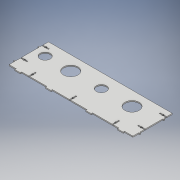
# Autodesk Inventor part: P1
Saved by Autodesk Inventor 2018 (Build 220112000, 112)
## iProperties
Created: 2018-02-28
Part Number: P1
Material: Generic
Document SubType Name: Modeling
Designer: isai
Density: 1 g/cm^3
Appearance: Default
Author: isai
Autodesk Inventor part; units mm, degrees
ref_plane "YZ Plane" through (0, 0, 0) normal (1, 0, 0) x (0, 1, 0)
sketch "Sketch2" plane through (0, 0, 0) normal (0, 0, 1) x (1, 0, 0)
  line L0 (220, -70) -> (-220, -70)
  line L1 (-220, -70) -> (-220, 70)
  line L2 (-220, 70) -> (220, 70)
  line L3 (220, 70) -> (220, -70)
  line L4 (220, -70) -> (-220, 70) construction
  line L5 (-220, -70) -> (220, 70) construction
  point P0 (0, 0)
  dimension "d8" = 440
  dimension "d9" = 140
  constraints: 12 end point, 2 midpoint, 2 parallel, 1 horizontal, 1 perpendicular
  measures "d8" distance of L1.end L2.end
  measures "d9" distance of L0.end L1.end
extrude "Extrusion2" add sketch "Sketch2" along normal blind 4
sketch "Sketch3" plane through (0, 0, 4) normal (0, 0, 1) x (1, 0, 0)
  line L0 (-220, -70) -> (220, -70) projected
  line L1 (220, -70) -> (220, 70) projected
  line L2 (220, 70) -> (-220, 70) projected
  line L3 (-220, 70) -> (-220, -70) projected
  circle A0 centre (-182, 20) radius 18
  circle A1 centre (-91, 20) radius 25.5
  circle A2 centre (18, 20) radius 18
  circle A3 centre (127, 20) radius 25.5
  point P0 (0, 0)
  dimension "d13" = 91
  dimension "d14" = 36
  dimension "d15" = 51
  dimension "d16" = 38
  dimension "d17" = 109
  dimension "d18" = 36
  dimension "d19" = 109
  dimension "d20" = 51
  dimension "d23" = 50
  constraints: 4 centre point, 2 coincident
  measures "d13" distance of A1.centre A0.centre
  measures "d14" diameter of A0
  measures "d15" diameter of A1
  measures "d16" distance from line of A0.centre L3
  measures "d17" distance of point (18, 20) A1.centre
  measures "d18" diameter of A2
  measures "d19" distance of point (127, 20) point (18, 20)
  measures "d20" diameter of A3
  measures "d23" distance from line of L2 A0.centre
extrude "Extrusion3" cut sketch "Sketch3" against normal blind 4 contours A0 | A1 | A2 | A3
sketch "Sketch4" plane through (0, 0, 4) normal (0, 0, 1) x (1, 0, 0)
  circle A0 centre (127, 20) radius 25.5
  circle A1 centre (18, 20) radius 25.5
  circle A2 centre (-91, 20) radius 18
  circle A3 centre (-182, 20) radius 18
  line L0 (-220, 70) -> (220, 70)
  line L1 (220, 70) -> (220, -70)
  line L2 (220, -70) -> (-220, -70)
  line L3 (-220, -70) -> (-220, 70)
  line L4 (220, 70) -> (224, 70)
  line L5 (224, -62.3) -> (220, -62.3)
  line L6 (224, 50) -> (197, 50)
  line L7 (197, 50) -> (197, 46.4)
  line L8 (197, 46.4) -> (224, 46.4)
  line L9 (224, 46.4) -> (224, 50)
  line L10 (210, 45.2) -> (207, 45.2)
  line L11 (207, 45.2) -> (207, 51.2)
  line L12 (207, 51.2) -> (210, 51.2)
  line L13 (210, 51.2) -> (210, 45.2)
  line L14 (210, 45.2) -> (207, 51.2) construction
  line L15 (207, 45.2) -> (210, 51.2) construction
  line L16 (224, -26.4) -> (197, -26.4)
  line L17 (197, -26.4) -> (197, -30)
  line L18 (197, -30) -> (224, -30)
  line L19 (224, -30) -> (224, -26.4)
  line L20 (210, -31.2) -> (207, -31.2)
  line L21 (207, -31.2) -> (207, -25.2)
  line L22 (207, -25.2) -> (210, -25.2)
  line L23 (210, -25.2) -> (210, -31.2)
  line L24 (210, -31.2) -> (207, -25.2) construction
  line L25 (207, -31.2) -> (210, -25.2) construction
  line L26 (224, 70) -> (224, 46.4)
  line L27 (224, -26.4) -> (224, -30)
  line L28 (220, -62.3) -> (220, -30)
  point P0 (0, 0)
  point P1 (208.5, 48.2)
  point P2 (208.5, -28.2)
  point P3 (220, 46.4)
  point P4 (220, -26.4)
  dimension "d24" = 4
  dimension "d25" = 27
  dimension "d26" = 3.6
  dimension "d27" = 3
  dimension "d28" = 6
  dimension "d29" = 10
  dimension "d30" = 140
  dimension "d31" = 20
  dimension "d32" = 27
  dimension "d33" = 3
  dimension "d34" = 6
  dimension "d35" = 40
  dimension "d36" = 3.6
  constraints: 58 end point, 11 parallel, 6 perpendicular, 5 horizontal, 4 centre point, 4 midpoint, 4 point on line
  measures "d24" distance of L5.start L28.start
  measures "d25" distance of L8.end L7.end
  measures "d26" distance of L7.end L6.end
  measures "d27" distance of L11.end L12.end
  measures "d28" distance of L10.end L11.end
  measures "d29" distance between parallel lines of L1 L13
  measures "d30" distance between parallel lines of L2 L0
  measures "d31" distance between parallel lines of L6 L0
  measures "d32" distance of L18.end L17.end
  measures "d33" distance of L22.start L22.end
  measures "d34" distance of L21.start L22.start
  measures "d35" distance between parallel lines of L2 L18
  measures "d36" distance of L17.start L17.end
extrude "Extrusion4" cut sketch "Sketch4" against normal blind 4 contours L6 L9 L8 L1 | L1 L8 L13 L6 | L13 L8 L11 L6 | L6 L11 L12 L13 | L16 L19 L18 L1 | L1 L18 L23 L16 | L13 L10 L11 L8 | L11 L8 L7 L6 | L23 L18 L21 L16 | L16 L21 L22 L23 | L23 L20 L21 L18 | L21 L18 L17 L16
ref_plane "Work Plane1" through (0, 70, 4) normal (1, 0, 0) x (0, 0, -1)
mirror "Mirror1" about plane through (0, 70, 4) normal (1, 0, 0) of "Extrusion4"
sketch "Sketch5" plane through (0, 0, 4) normal (0, 0, 1) x (1, 0, 0)
  line L0 (-224, -46) -> (-220, -46)
  line L1 (-224, -50) -> (-224, -46)
  line L2 (-220, -50) -> (-224, -50)
  line L3 (-220, -50) -> (-220, -70)
  line L4 (-220, -70) -> (220, -70)
  line L5 (220, -70) -> (220, -50)
  line L6 (220, -50) -> (224, -50)
  line L7 (224, -50) -> (224, -46)
  line L8 (224, -46) -> (220, -46)
  line L9 (-150, -57) -> (-150, -47)
  line L10 (-151.2, -57) -> (-150, -57)
  line L11 (-150, -47) -> (-146.4, -47)
  line L12 (-146.4, -47) -> (-146.4, -57)
  line L13 (-146.4, -57) -> (-145.2, -57)
  line L14 (-150, -60) -> (-151.2, -60)
  line L15 (-151.2, -60) -> (-151.2, -57)
  line L16 (-145.2, -57) -> (-145.2, -60)
  line L17 (-145.2, -60) -> (-146.4, -60)
  line L18 (-150, -70) -> (-150, -60)
  line L19 (-146.4, -60) -> (-146.4, -70)
  line L20 (-146.4, -70) -> (-150, -70)
  line L21 (-220, -70) -> (220, -70)
  line L22 (151.2, -57) -> (151.2, -60)
  line L23 (150, -57) -> (151.2, -57)
  line L24 (150, -47) -> (150, -57)
  line L25 (146.4, -47) -> (150, -47)
  line L26 (150, -60) -> (150, -70)
  line L27 (146.4, -57) -> (146.4, -47)
  line L28 (146.4, -70) -> (146.4, -60)
  line L29 (145.2, -57) -> (146.4, -57)
  line L30 (145.2, -60) -> (145.2, -57)
  line L31 (146.4, -60) -> (145.2, -60)
  line L32 (151.2, -60) -> (150, -60)
  line L33 (150, -70) -> (146.4, -70)
  line L34 (-0.6, -57) -> (-0.6, -60)
  line L35 (-1.8, -57) -> (-0.6, -57)
  line L36 (-1.8, -47) -> (-1.8, -57)
  line L37 (-5.4, -47) -> (-1.8, -47)
  line L38 (-1.8, -60) -> (-1.8, -70)
  line L39 (-5.4, -57) -> (-5.4, -47)
  line L40 (-5.4, -70) -> (-5.4, -60)
  line L41 (-6.6, -57) -> (-5.4, -57)
  line L42 (-6.6, -60) -> (-6.6, -57)
  line L43 (-5.4, -60) -> (-6.6, -60)
  line L44 (-0.6, -60) -> (-1.8, -60)
  line L45 (-1.8, -70) -> (-5.4, -70)
  line L46 (-220, -70) -> (220, -70) projected
  point P0 (0, 0)
  point P1 (-143.2198, -70)
  point P2 (176.1378, -65.3908)
  point P3 (10.9651, -65.3908)
  dimension "d39" = 70
  dimension "d40" = 3.6
  dimension "d41" = 3.6
  dimension "d42" = 6
  dimension "d43" = 1.2
  dimension "d44" = 3
  dimension "d45" = 1.2
  dimension "d46" = 3.6
  dimension "d47" = 3.6
  dimension "d48" = 6
  dimension "d49" = 1.2
  dimension "d50" = 3
  dimension "d51" = 1.2
  dimension "d52" = 3.6
  dimension "d53" = 3.6
  dimension "d54" = 6
  dimension "d55" = 1.2
  dimension "d56" = 3
  dimension "d57" = 1.2
  dimension "d58" = 70
  dimension "d59" = 440
  dimension "d60" = 221.8
  constraints: 92 end point, 18 perpendicular, 3 parallel, 1 point on line
  measures "d39" distance between parallel lines of L18 L3
  measures "d40" distance between parallel lines of L19 L18
  measures "d41" distance between parallel lines of L12 L9
  measures "d42" distance between parallel lines of L16 L15
  measures "d43" distance between parallel lines of L15 L9
  measures "d44" distance between parallel lines of L14 L10
  measures "d45" distance between parallel lines of L18 L15
  measures "d46" distance between parallel lines of L26 L28
  measures "d47" distance between parallel lines of L24 L27
  measures "d48" distance between parallel lines of L22 L30
  measures "d49" distance between parallel lines of L30 L27
  measures "d50" distance between parallel lines of L31 L29
  measures "d51" distance between parallel lines of L28 L30
  measures "d52" distance between parallel lines of L38 L40
  measures "d53" distance between parallel lines of L36 L39
  measures "d54" distance between parallel lines of L34 L42
  measures "d55" distance between parallel lines of L42 L39
  measures "d56" distance between parallel lines of L43 L41
  measures "d57" distance between parallel lines of L40 L42
  measures "d58" distance between parallel lines of L5 L26
  measures "d59" distance between parallel lines of L5 L3
  measures "d60" distance between parallel lines of L5 L38
extrude "Extrusion5" cut sketch "Sketch5" against normal blind 10
sketch "Sketch6" plane through (0, 0, 4) normal (0, 0, 1) x (1, 0, 0)
  line L0 (-220, -70) -> (-150, -70)
  line L1 (-195, -70) -> (-175, -70)
  line L2 (-175, -70) -> (-175, -75)
  line L3 (-175, -75) -> (-195, -75)
  line L4 (-195, -75) -> (-195, -70)
  line L5 (-146.4, -70) -> (-5.4, -70)
  line L6 (-85.9, -70) -> (-65.9, -70)
  line L7 (-65.9, -70) -> (-65.9, -75)
  line L8 (-65.9, -75) -> (-85.9, -75)
  line L9 (-85.9, -75) -> (-85.9, -70)
  line L10 (-1.8, -70) -> (146.4, -70)
  line L11 (57.1516, -70) -> (77.1516, -70)
  line L12 (77.1516, -70) -> (77.1516, -75)
  line L13 (77.1516, -75) -> (57.1516, -75)
  line L14 (57.1516, -75) -> (57.1516, -70)
  line L15 (150, -70) -> (220, -70)
  line L16 (170.4397, -70) -> (190.4397, -70)
  line L17 (190.4397, -70) -> (190.4397, -75)
  line L18 (190.4397, -75) -> (170.4397, -75)
  line L19 (170.4397, -75) -> (170.4397, -70)
  line L20 (-220, -50) -> (-220, -70)
  line L21 (-146.4, -60) -> (-146.4, -70)
  line L22 (-5.4, -70) -> (-5.4, -60)
  line L23 (146.4, -70) -> (146.4, -60)
  line L24 (-1.8, -60) -> (-1.8, -70)
  line L25 (-1.8, -60) -> (-1.8, -70) projected
  line L26 (-1.8, -70) -> (146.4, -70) projected
  line L27 (146.4, -70) -> (146.4, -60) projected
  line L28 (146.4, -60) -> (145.2, -60) projected
  line L29 (145.2, -60) -> (145.2, -57) projected
  line L30 (145.2, -57) -> (146.4, -57) projected
  line L31 (146.4, -57) -> (146.4, -47) projected
  line L32 (146.4, -47) -> (150, -47) projected
  line L33 (150, -47) -> (150, -57) projected
  line L34 (150, -57) -> (151.2, -57) projected
  line L35 (151.2, -57) -> (151.2, -60) projected
  line L36 (151.2, -60) -> (150, -60) projected
  line L37 (150, -60) -> (150, -70) projected
  line L38 (150, -70) -> (220, -70) projected
  line L39 (220, -70) -> (220, -30) projected
  line L40 (220, -30) -> (210, -30) projected
  line L41 (210, -30) -> (210, -31.2) projected
  line L42 (210, -31.2) -> (207, -31.2) projected
  line L43 (207, -31.2) -> (207, -30) projected
  line L44 (207, -30) -> (197, -30) projected
  line L45 (197, -30) -> (197, -26.4) projected
  line L46 (197, -26.4) -> (207, -26.4) projected
  line L47 (207, -26.4) -> (207, -25.2) projected
  line L48 (207, -25.2) -> (210, -25.2) projected
  line L49 (210, -25.2) -> (210, -26.4) projected
  line L50 (210, -26.4) -> (220, -26.4) projected
  line L51 (220, -26.4) -> (220, 46.4) projected
  line L52 (220, 46.4) -> (210, 46.4) projected
  line L53 (210, 46.4) -> (210, 45.2) projected
  line L54 (210, 45.2) -> (207, 45.2) projected
  line L55 (207, 45.2) -> (207, 46.4) projected
  line L56 (207, 46.4) -> (197, 46.4) projected
  line L57 (197, 46.4) -> (197, 50) projected
  line L58 (197, 50) -> (207, 50) projected
  line L59 (207, 50) -> (207, 51.2) projected
  line L60 (207, 51.2) -> (210, 51.2) projected
  line L61 (210, 51.2) -> (210, 50) projected
  line L62 (210, 50) -> (220, 50) projected
  line L63 (220, 50) -> (220, 70) projected
  line L64 (220, 70) -> (-220, 70) projected
  line L65 (-220, 70) -> (-220, 50) projected
  line L66 (-220, 50) -> (-210, 50) projected
  line L67 (-210, 50) -> (-210, 51.2) projected
  line L68 (-210, 51.2) -> (-207, 51.2) projected
  line L69 (-207, 51.2) -> (-207, 50) projected
  line L70 (-207, 50) -> (-197, 50) projected
  line L71 (-197, 50) -> (-197, 46.4) projected
  line L72 (-197, 46.4) -> (-207, 46.4) projected
  line L73 (-207, 46.4) -> (-207, 45.2) projected
  line L74 (-207, 45.2) -> (-210, 45.2) projected
  line L75 (-210, 45.2) -> (-210, 46.4) projected
  line L76 (-210, 46.4) -> (-220, 46.4) projected
  line L77 (-220, 46.4) -> (-220, -26.4) projected
  line L78 (-220, -26.4) -> (-210, -26.4) projected
  line L79 (-210, -26.4) -> (-210, -25.2) projected
  line L80 (-210, -25.2) -> (-207, -25.2) projected
  line L81 (-207, -25.2) -> (-207, -26.4) projected
  line L82 (-207, -26.4) -> (-197, -26.4) projected
  line L83 (-197, -26.4) -> (-197, -30) projected
  line L84 (-197, -30) -> (-207, -30) projected
  line L85 (-207, -30) -> (-207, -31.2) projected
  line L86 (-207, -31.2) -> (-210, -31.2) projected
  line L87 (-210, -31.2) -> (-210, -30) projected
  line L88 (-210, -30) -> (-220, -30) projected
  line L89 (-220, -30) -> (-220, -70) projected
  line L90 (-220, -70) -> (-150, -70) projected
  line L91 (-150, -70) -> (-150, -60) projected
  line L92 (-150, -60) -> (-151.2, -60) projected
  line L93 (-151.2, -60) -> (-151.2, -57) projected
  line L94 (-151.2, -57) -> (-150, -57) projected
  line L95 (-150, -57) -> (-150, -47) projected
  line L96 (-150, -47) -> (-146.4, -47) projected
  line L97 (-146.4, -47) -> (-146.4, -57) projected
  line L98 (-146.4, -57) -> (-145.2, -57) projected
  line L99 (-145.2, -57) -> (-145.2, -60) projected
  line L100 (-145.2, -60) -> (-146.4, -60) projected
  line L101 (-146.4, -60) -> (-146.4, -70) projected
  line L102 (-146.4, -70) -> (-5.4, -70) projected
  line L103 (-5.4, -70) -> (-5.4, -60) projected
  line L104 (-5.4, -60) -> (-6.6, -60) projected
  line L105 (-6.6, -60) -> (-6.6, -57) projected
  line L106 (-6.6, -57) -> (-5.4, -57) projected
  line L107 (-5.4, -57) -> (-5.4, -47) projected
  line L108 (-5.4, -47) -> (-1.8, -47) projected
  line L109 (-1.8, -47) -> (-1.8, -57) projected
  line L110 (-1.8, -57) -> (-0.6, -57) projected
  line L111 (-0.6, -57) -> (-0.6, -60) projected
  line L112 (-0.6, -60) -> (-1.8, -60) projected
  circle A0 centre (-91, 20) radius 25.5 projected
  circle A1 centre (-182, 20) radius 18 projected
  circle A2 centre (18, 20) radius 18 projected
  circle A3 centre (127, 20) radius 25.5 projected
  line L113 (-220, -30) -> (-220, -70) projected
  point P0 (0, 0)
  dimension "d63" = 20
  dimension "d64" = 5
  dimension "d65" = 20
  dimension "d66" = 5
  dimension "d67" = 20
  dimension "d68" = 5
  dimension "d69" = 20
  dimension "d70" = 5
  dimension "d71" = 25
  dimension "d72" = 60.5
  dimension "d73" = 141
  dimension "d74" = 148.2
  constraints: 50 end point, 8 parallel, 4 horizontal, 4 perpendicular, 4 point on line, 2 coincident
  measures "d63" distance of L2.end L3.end
  measures "d64" distance of L2.start L2.end
  measures "d65" distance of L7.end L9.start
  measures "d66" distance of L6.end L7.end
  measures "d67" distance of L12.end L14.start
  measures "d68" distance of L12.start L12.end
  measures "d69" distance of L17.end L19.start
  measures "d70" distance of L17.start L17.end
  measures "d71" distance between parallel lines of L4 L20
  measures "d72" distance between parallel lines of L9 L21
  measures "d73" distance between parallel lines of L22 L21
  measures "d74" distance between parallel lines of L23 L24
extrude "Extrusion6" add sketch "Sketch6" against normal blind 4 contours L0 L2 L3 L4 | L5 L7 L8 L9 | L10 L12 L13 L14 | L15 L17 L18 L19
sketch "Sketch7" plane through (0, 0, 4) normal (0, 0, 1) x (1, 0, 0)
  line L0 (220, 70) -> (-220, 70)
  line L1 (210, -26.4) -> (220, -26.4)
  line L2 (220, -26.4) -> (220, 46.4)
  line L3 (220, 46.4) -> (210, 46.4)
  line L4 (210, 46.4) -> (210, 45.2)
  line L5 (210, 45.2) -> (207, 45.2)
  line L6 (207, 45.2) -> (207, 46.4)
  line L7 (207, 46.4) -> (197, 46.4)
  line L8 (197, 50) -> (207, 50)
  line L9 (207, 50) -> (207, 51.2)
  line L10 (207, 51.2) -> (210, 51.2)
  line L11 (210, 51.2) -> (210, 50)
  line L12 (210, 50) -> (220, 50)
  line L13 (220, 50) -> (220, 70)
  line L14 (220, 70) -> (-220, 70)
  line L15 (-220, -70) -> (220, -70)
  line L16 (220, -70) -> (220, -30)
  line L17 (220, -30) -> (210, -30)
  line L18 (210, -30) -> (210, -31.2)
  line L19 (210, -31.2) -> (207, -31.2)
  line L20 (207, -31.2) -> (207, -30)
  line L21 (207, -30) -> (197, -30)
  line L22 (197, -26.4) -> (207, -26.4)
  line L23 (207, -26.4) -> (207, -25.2)
  line L24 (207, -25.2) -> (210, -25.2)
  line L25 (210, -25.2) -> (210, -26.4)
  circle A0 centre (182, 20) radius 18
  line L26 (220, 40) -> (224, 40)
  line L27 (224, 40) -> (224, 36)
  line L28 (224, 36) -> (220, 36)
  line L29 (220, 36) -> (220, 40)
  line L30 (220, -46) -> (224, -46)
  line L31 (224, -46) -> (224, -50)
  line L32 (224, -50) -> (220, -50)
  line L33 (220, -50) -> (220, -46)
  line L34 (-1.8, -60) -> (-1.8, -70) projected
  line L35 (-1.8, -70) -> (57.1516, -70) projected
  line L36 (57.1516, -70) -> (57.1516, -75) projected
  line L37 (57.1516, -75) -> (77.1516, -75) projected
  line L38 (77.1516, -75) -> (77.1516, -70) projected
  line L39 (77.1516, -70) -> (146.4, -70) projected
  line L40 (146.4, -70) -> (146.4, -60) projected
  line L41 (146.4, -60) -> (145.2, -60) projected
  line L42 (145.2, -60) -> (145.2, -57) projected
  line L43 (145.2, -57) -> (146.4, -57) projected
  line L44 (146.4, -57) -> (146.4, -47) projected
  line L45 (146.4, -47) -> (150, -47) projected
  line L46 (150, -47) -> (150, -57) projected
  line L47 (150, -57) -> (151.2, -57) projected
  line L48 (151.2, -57) -> (151.2, -60) projected
  line L49 (151.2, -60) -> (150, -60) projected
  line L50 (150, -60) -> (150, -70) projected
  line L51 (150, -70) -> (170.4397, -70) projected
  line L52 (170.4397, -75) -> (170.4397, -70) projected
  line L53 (190.4397, -75) -> (170.4397, -75) projected
  line L54 (190.4397, -70) -> (190.4397, -75) projected
  line L55 (190.4397, -70) -> (220, -70) projected
  line L56 (220, -70) -> (220, -30) projected
  line L57 (220, -30) -> (210, -30) projected
  line L58 (210, -30) -> (210, -31.2) projected
  line L59 (210, -31.2) -> (207, -31.2) projected
  line L60 (207, -31.2) -> (207, -30) projected
  line L61 (207, -30) -> (197, -30) projected
  line L62 (197, -30) -> (197, -26.4) projected
  line L63 (197, -26.4) -> (207, -26.4) projected
  line L64 (207, -26.4) -> (207, -25.2) projected
  line L65 (207, -25.2) -> (210, -25.2) projected
  line L66 (210, -25.2) -> (210, -26.4) projected
  line L67 (210, -26.4) -> (220, -26.4) projected
  line L68 (220, -26.4) -> (220, 46.4) projected
  line L69 (220, 46.4) -> (210, 46.4) projected
  line L70 (210, 46.4) -> (210, 45.2) projected
  line L71 (210, 45.2) -> (207, 45.2) projected
  line L72 (207, 45.2) -> (207, 46.4) projected
  line L73 (207, 46.4) -> (197, 46.4) projected
  line L74 (197, 46.4) -> (197, 50) projected
  line L75 (197, 50) -> (207, 50) projected
  line L76 (207, 50) -> (207, 51.2) projected
  line L77 (207, 51.2) -> (210, 51.2) projected
  line L78 (210, 51.2) -> (210, 50) projected
  line L79 (210, 50) -> (220, 50) projected
  line L80 (220, 50) -> (220, 70) projected
  line L81 (220, 70) -> (-220, 70) projected
  line L82 (-220, 70) -> (-220, 50) projected
  line L83 (-220, 50) -> (-210, 50) projected
  line L84 (-210, 50) -> (-210, 51.2) projected
  line L85 (-210, 51.2) -> (-207, 51.2) projected
  line L86 (-207, 51.2) -> (-207, 50) projected
  line L87 (-207, 50) -> (-197, 50) projected
  line L88 (-197, 50) -> (-197, 46.4) projected
  line L89 (-197, 46.4) -> (-207, 46.4) projected
  line L90 (-207, 46.4) -> (-207, 45.2) projected
  line L91 (-207, 45.2) -> (-210, 45.2) projected
  line L92 (-210, 45.2) -> (-210, 46.4) projected
  line L93 (-210, 46.4) -> (-220, 46.4) projected
  line L94 (-220, 46.4) -> (-220, -26.4) projected
  line L95 (-220, -26.4) -> (-210, -26.4) projected
  line L96 (-210, -26.4) -> (-210, -25.2) projected
  line L97 (-210, -25.2) -> (-207, -25.2) projected
  line L98 (-207, -25.2) -> (-207, -26.4) projected
  line L99 (-207, -26.4) -> (-197, -26.4) projected
  line L100 (-197, -26.4) -> (-197, -30) projected
  line L101 (-197, -30) -> (-207, -30) projected
  line L102 (-207, -30) -> (-207, -31.2) projected
  line L103 (-207, -31.2) -> (-210, -31.2) projected
  line L104 (-210, -31.2) -> (-210, -30) projected
  line L105 (-210, -30) -> (-220, -30) projected
  line L106 (-220, -30) -> (-220, -70) projected
  line L107 (-220, -70) -> (-195, -70) projected
  line L108 (-195, -70) -> (-195, -75) projected
  line L109 (-195, -75) -> (-175, -75) projected
  line L110 (-175, -75) -> (-175, -70) projected
  line L111 (-175, -70) -> (-150, -70) projected
  line L112 (-150, -70) -> (-150, -60) projected
  line L113 (-150, -60) -> (-151.2, -60) projected
  line L114 (-151.2, -60) -> (-151.2, -57) projected
  line L115 (-151.2, -57) -> (-150, -57) projected
  line L116 (-150, -57) -> (-150, -47) projected
  line L117 (-150, -47) -> (-146.4, -47) projected
  line L118 (-146.4, -47) -> (-146.4, -57) projected
  line L119 (-146.4, -57) -> (-145.2, -57) projected
  line L120 (-145.2, -57) -> (-145.2, -60) projected
  line L121 (-145.2, -60) -> (-146.4, -60) projected
  line L122 (-146.4, -60) -> (-146.4, -70) projected
  line L123 (-146.4, -70) -> (-85.9, -70) projected
  line L124 (-85.9, -70) -> (-85.9, -75) projected
  line L125 (-85.9, -75) -> (-65.9, -75) projected
  line L126 (-65.9, -75) -> (-65.9, -70) projected
  line L127 (-65.9, -70) -> (-5.4, -70) projected
  line L128 (-5.4, -70) -> (-5.4, -60) projected
  line L129 (-5.4, -60) -> (-6.6, -60) projected
  line L130 (-6.6, -60) -> (-6.6, -57) projected
  line L131 (-6.6, -57) -> (-5.4, -57) projected
  line L132 (-5.4, -57) -> (-5.4, -47) projected
  line L133 (-5.4, -47) -> (-1.8, -47) projected
  line L134 (-1.8, -47) -> (-1.8, -57) projected
  line L135 (-1.8, -57) -> (-0.6, -57) projected
  line L136 (-0.6, -57) -> (-0.6, -60) projected
  line L137 (-0.6, -60) -> (-1.8, -60) projected
  circle A1 centre (-91, 20) radius 25.5 projected
  circle A2 centre (-182, 20) radius 18 projected
  circle A3 centre (18, 20) radius 18 projected
  circle A4 centre (127, 20) radius 25.5 projected
  line L138 (-220, -70) -> (-220, -30) projected
  point P0 (0, 0)
  dimension "d77" = 4
  dimension "d78" = 4
  dimension "d79" = 4
  dimension "d80" = 4
  dimension "d81" = 20
  dimension "d82" = 30
  constraints: 68 end point, 4 parallel, 2 horizontal, 2 perpendicular, 2 point on line, 1 centre point, 1 coincident
  measures "d77" distance of L27.end L29.start
  measures "d78" distance of L27.start L27.end
  measures "d79" distance of L31.end L33.start
  measures "d80" distance of L30.end L31.end
  measures "d81" distance between parallel lines of L32 L15
  measures "d82" distance between parallel lines of L26 L0
extrude "Extrusion7" add sketch "Sketch7" against normal blind 4 contours L26 L27 L28 L2 | L30 L31 L32 L16
ref_plane "Work Plane2" through (0, -26.4, 4) normal (1, 0, 0) x (0, 0, -1)
mirror "Mirror2" about plane through (0, -26.4, 4) normal (1, 0, 0) of "Extrusion7"
body "Solid2"
